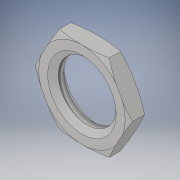
# Autodesk Inventor part: AT513H
Saved by Autodesk Inventor 2019 (Build 230136000, 136)
## iProperties
Created: 2022-08-22
Part Number: AT513H
Material: Generic
Catalog Web Link: www.cadenas.de
Description: Hex Nut - Bushing Mount Miniature Toggles-Series M - Standard Hardwarw for Small & Large Bushings
Vendor: NKKSWITCHES
Document SubType Name: Modeling
Designer: psAdmin
Manufacturer: NKKSWITCHES
Mass: 0.0428017 g
Surface Area: 1.17936 cm^2
Volume: 0.0428017 cm^3
Density: 1 g/cm^3
Appearance: PSOLRGB-175-175-175
Category: PARTsolutions
Company: NKKSWITCHES
Title: AT513H
Author: Cadenas PARTsolutions
Comments: Series M - Standard Hardwarw for Small & Large Bushings
PSOL_IDENT_0: {$CADENAS_DATA/23d-libs/nkkswitches/toggle/m/hardware/hex_nut.prj},187 {VTYP=3D},{NB=AT513H},{LINA=A
PSOL_IDENT_1: T513H},{NN=Hex Nut - Bushing Mount Miniature Toggles},{DATE=02.08.2022 07:27:08},{GEOMDATE=07.12.200
PSOL_IDENT_2: 9 11:39:00},{VERSION=},{LINEID=10},{WBVAR=},{WBNUMERIC=}  {NB=AT513H},{LINA=AT513H},{KT=DUMMY},{PN=A
PSOL_IDENT_3: T513H},{S=0.315},{D=1/4-40},{DMAX=0.25},{DMIN=0.22},{T=0.059},{W=0.354}
NB: AT513H
NN: Hex Nut - Bushing Mount Miniature Toggles
NT: Series M - Standard Hardwarw for Small & Large Bushings
NBSYN: $PN.
LINA: AT513H
CATALOG: NKK Switches
PN: AT513H
S: 0.315
D: 1/4-40
T: 0.059
W: 0.354
SUPPLIER: NKKSWITCHES
ARTICLENO: AT513H
BOMINFO: AT513H
CREATOR: CADENAS GmbH
Autodesk Inventor part; units mm, degrees
sketch "Sketch_1" plane through (0, 0, 0) normal (1, 0, 0) x (0, 1, 0)
  line L0 (0, -0.7493) -> (0, 0.7493)
  line L1 (0, 0.7493) -> (4.0005, 0.7493)
  line L2 (4.0005, 0.7493) -> (4.8006, 0.4581)
  line L3 (4.8006, 0.4581) -> (4.8006, -0.4581)
  line L4 (4.8006, -0.4581) -> (4.0005, -0.7493)
  line L5 (4.0005, -0.7493) -> (0, -0.7493)
  line L6 (0, -0.7493) -> (0, 0.7493)
  constraints: 14 end point
revolve "Revolution1" add sketch "Sketch_1" angle 360 about axis through (0, 0, -0.7493) along (0, 0, -1)
sketch "Sketch_2" plane through (0, 0, 0) normal (0, 0, 1) x (1, 0, 0)
  line L0 (-8.001, -8.001) -> (8.001, -8.001)
  line L1 (8.001, -8.001) -> (8.001, 8.001)
  line L2 (8.001, 8.001) -> (-8.001, 8.001)
  line L3 (-8.001, 8.001) -> (-8.001, -8.001)
  line L4 (-4.4958, 0) -> (-2.3097, -4.0005)
  line L5 (-2.3097, -4.0005) -> (2.3097, -4.0005)
  line L6 (2.3097, -4.0005) -> (4.4958, 0)
  line L7 (4.4958, 0) -> (2.3097, 4.0005)
  line L8 (2.3097, 4.0005) -> (-2.3097, 4.0005)
  line L9 (-2.3097, 4.0005) -> (-4.4958, 0)
  constraints: 20 end point
extrude "Extrusion1" cut sketch "Sketch_2" along normal mid plane 2.9972
sketch "Sketch_6" plane through (0, 0, 0) normal (1, 0, 0) x (0, 1, 0)
  line L0 (0, -0.7493) -> (0, 0.7493)
  line L1 (0, 0.7493) -> (3.175, 0.7493)
  line L2 (3.175, 0.7493) -> (2.6835, 0.2578)
  line L3 (2.6835, 0.2578) -> (2.6835, -0.2578)
  line L4 (2.6835, -0.2578) -> (3.175, -0.7493)
  line L5 (3.175, -0.7493) -> (0, -0.7493)
  line L6 (0, -0.7493) -> (0, 0.7493)
  constraints: 14 end point
revolve "Revolution2" cut sketch "Sketch_6" angle 360 about axis through (0, 0, -0.7493) along (0, 0, -1)
thread "Thread1" size "1/4-28 UNF" class "2B" standard "ANSI Unified Screw Threads" full length
ref_plane "nut_XY" through (0, 0, 0.7493) normal (0, 0, 1) x (1, 0, 0)
ref_plane "nut_YZ" through (0, 0, 0.7493) normal (1, 0, 0) x (0, 1, 0)
ref_plane "nut_ZX" through (0, 0, 0.7493) normal (0, 1, 0) x (0, 0, 1)
body "Solid1"
